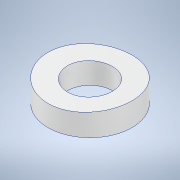
# Autodesk Inventor part: Spacers
Saved by Autodesk Inventor 2021 (Build 250183000, 183)
## iProperties
Created: 2021-10-19
Part Number: Spacers
Material: Aluminum 6061
Document SubType Name: Modeling
Designer: Alex Clay
Density: 2.7 g/cm^3
Appearance: Aluminum - Flat
Mass: 0.806139 g
Surface Area: 3.83925 cm^2
Volume: 0.29857 cm^3
Author: Alex Clay
Autodesk Inventor part; units mm, degrees
ref_plane "YZ Plane" through (0, 0, 0) normal (1, 0, 0) x (0, 1, 0)
ref_plane "XZ Plane" through (0, 0, 0) normal (0, 1, 0) x (-1, 0, 0)
ref_plane "XY Plane" through (0, 0, 0) normal (0, 0, 1) x (1, 0, 0)
sketch "Sketch1" plane through (0, 0, 0) normal (0, 1, 0) x (-1, 0, 0)
  circle A0 centre (0, 0) radius 6.35
  dimension "d0" = 12.7
  constraints: 1 centre point, 1 coincident
  measures "d0" diameter of A0
extrude "Extrusion1" add sketch "Sketch1" along normal blind 12.7
sketch "Sketch2" plane through (0, 0, 0) normal (0, 0, 1) x (1, 0, 0)
  circle A0 centre (0, 60.325) radius 57.15
  line L0 (-41.9347, 3.175) -> (51.5907, 3.175) construction
  point P0 (0, 0)
  dimension "d3" = 114.3
  dimension "d4" = 3.175
  constraints: 2 end point, 1 centre point, 1 horizontal, 1 tangent, 1 vertical alignment
  measures "d3" diameter of A0
  measures "d4" distance from line of point (0, 0) L0
extrude "Extrusion2" cut sketch "Sketch2" along normal through all both and the other way through all
sketch "Sketch4" plane through (0, 0, 0) normal (0, -1, 0) x (1, 0, 0)
  point P0 (0, 0)
  point P1 (0, 0)
  constraints: 1 coincident
hole "Hole1" at (0, 0, 0) direction (0, 1, 0) diameter 6.7564 end through all clearance for "Socket Head Cap Screw" size "1/4" standard "Ansi Unified Screw Threads"
body "Solid1"
